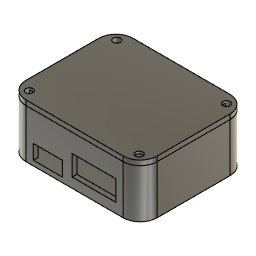
Box_motor (Autodesk Fusion 360 design; units mm, degrees)
Autodesk Fusion 360 part; units mm, degrees
sketch "Sketch1" plane through (0, 0, 0) normal (0, 0, 1) x (1, 0, 0)
  line L0 (-20, 20) -> (20, 20)
  line L1 (25, 15) -> (25, -15)
  line L2 (20, -20) -> (-20, -20)
  line L3 (-25, -15) -> (-25, 15)
  line L4 (-25, 20) -> (25, -20) construction
  line L5 (25, 20) -> (-25, -20) construction
  arc A0 (-25, -15) -> (-20, -20) centre (-20, -15) ccw
  arc A1 (-20, 20) -> (-25, 15) centre (-20, 15) ccw
  arc A2 (25, 15) -> (20, 20) centre (20, 15) ccw
  arc A3 (20, -20) -> (25, -15) centre (20, -15) ccw
  line L6 (20, -22) -> (-20, -22)
  arc A4 (-27, -15) -> (-20, -22) centre (-20, -15) ccw
  line L7 (-27, -15) -> (-27, 15)
  arc A5 (-20, 22) -> (-27, 15) centre (-20, 15) ccw
  line L8 (-20, 22) -> (20, 22)
  arc A6 (27, 15) -> (20, 22) centre (20, 15) ccw
  line L9 (27, 15) -> (27, -15)
  arc A7 (20, -22) -> (27, -15) centre (20, -15) ccw
  dimension "d1" = 50
  dimension "d2" = 40
  dimension "d3" = -2
  dimension "d4" = 5
  dimension "d5" = 5
  constraint horizontal L0
  constraint perpendicular L0 L1
  constraint parallel L0 L2
  constraint parallel L1 L3
  constraint coincident L4 origin
  constraint coincident L5 origin
  constraint coincident L5.end L3
  constraint coincident L5.end L2
  constraint tangent L3 A0
  constraint tangent L2 A0
  constraint coincident L4.start L3
  constraint coincident L4.start L0
  constraint tangent L3 A1
  constraint tangent L0 A1
  constraint equal A0 A1
  constraint coincident L5.start L1
  constraint coincident L5.start L0
  constraint tangent L1 A2
  constraint tangent L0 A2
  constraint coincident L4.end L1
  constraint coincident L4.end L2
  constraint tangent L1 A3
  constraint tangent L2 A3
  constraint equal A2 A3
  measures "d1" distance of L4.end L5.end
  measures "d2" distance of L5.start L4.end
  measures "d4" radius of A0
  measures "d5" radius of A2
extrude "Extrude1" add sketch "Sketch1" along normal blind 20 contours L0 L1 L2 L3 A0 A1 A2 A3 | L6 A4 L7 A5 L8 A6 L9 A7 makes body 1
shell "Shell1" thickness 2 removed faces 1 at (6.6667, -7.3333, 20) on bodies 1
sketch "Sketch2" plane through (0, -22, 0) normal (0, -1, 0) x (1, 0, 0)
  line L0 (-20, 0) -> (20, 0)
  line L1 (20, 0) -> (20, 20)
  line L2 (20, 20) -> (-20, 20)
  line L3 (-20, 20) -> (-20, 0)
  line L4 (-17, 8) -> (-5, 8)
  line L5 (-5, 8) -> (-5, 2)
  line L6 (-5, 2) -> (-17, 2)
  line L7 (-17, 2) -> (-17, 8)
  line L8 (-27, 0) -> (-27, 20)
  line L9 (-1, 2) -> (17, 2)
  line L10 (17, 2) -> (17, 12.4065)
  line L11 (17, 12.4065) -> (-1, 12.4065)
  line L12 (-1, 12.4065) -> (-1, 2)
  dimension "d9" = 10
  dimension "d10" = 12
  dimension "d11" = 2
  dimension "d12" = 6
  dimension "d13" = 2
  dimension "d14" = 4
  dimension "d15" = 18
  constraint horizontal L4
  constraint vertical L5
  constraint horizontal L6
  constraint vertical L7
  constraint horizontal L9
  constraint vertical L10
  constraint horizontal L11
  constraint vertical L12
  measures "d9" distance of L7 L8
  measures "d10" distance of L4.start L4.end
  measures "d11" distance of L0 L6
  measures "d12" distance of L4.end L5.end
  measures "d13" distance of L0 L9
  measures "d14" distance of L5 L12
  measures "d15" distance of L10.end L11.end
extrude "Extrude2" cut sketch "Sketch2" against normal blind 10 contours L4 L5 L6 L7 | L9 L10 L11 L12 bodies 1
sketch "Sketch3" plane through (0, 0, 20) normal (0, 0, 1) x (-1, 0, 0)
  line L0 (25, 15) -> (25, -15)
  arc A0 (20, -20) -> (25, -15) centre (20, -15) ccw
  line L1 (20, -20) -> (-20, -20)
  arc A1 (-25, -15) -> (-20, -20) centre (-20, -15) ccw
  line L2 (-25, -15) -> (-25, 15)
  arc A2 (-20, 20) -> (-25, 15) centre (-20, 15) ccw
  line L3 (-20, 20) -> (20, 20)
  arc A3 (25, 15) -> (20, 20) centre (20, 15) ccw
  arc A4 (27, 15) -> (20, 22) centre (20, 15) ccw
  line L4 (20, 22) -> (-20, 22)
  arc A5 (-20, 22) -> (-27, 15) centre (-20, 15) ccw
  line L5 (-27, 15) -> (-27, -15)
  arc A6 (-27, -15) -> (-20, -22) centre (-20, -15) ccw
  line L6 (-20, -22) -> (20, -22)
  arc A7 (20, -22) -> (27, -15) centre (20, -15) ccw
  line L7 (27, -15) -> (27, 15)
extrude "Extrude3" add sketch "Sketch3" along normal blind 2 separate body contours L0 A0 L1 A1 L2 A2 L3 A3 | A4 L4 A5 L5 A6 L6 A7 L7 makes body 2
extrude "Extrude4" add sketch "Sketch3" against normal blind 2 contours L0 A0 L1 A1 L2 A2 L3 A3 bodies 2
shell "Shell2" thickness 1 removed faces 1 at (6.6667, -6.6667, 18) on bodies 2
sketch "Sketch4" plane through (0, 0, 20) normal (0, 0, 1) x (-1, 0, 0)
  line L0 (25, 15) -> (25, -15)
  arc A0 (20, -20) -> (25, -15) centre (20, -15) ccw
  line L1 (20, -20) -> (-20, -20)
  arc A1 (-25, -15) -> (-20, -20) centre (-20, -15) ccw
  line L2 (-25, -15) -> (-25, 15)
  arc A2 (-20, 20) -> (-25, 15) centre (-20, 15) ccw
  line L3 (-20, 20) -> (20, 20)
  arc A3 (25, 15) -> (20, 20) centre (20, 15) ccw
  arc A4 (27, 15) -> (20, 22) centre (20, 15) ccw
  line L4 (20, 22) -> (-20, 22)
  arc A5 (-20, 22) -> (-27, 15) centre (-20, 15) ccw
  line L5 (-27, 15) -> (-27, -15)
  arc A6 (-27, -15) -> (-20, -22) centre (-20, -15) ccw
  line L6 (-20, -22) -> (20, -22)
  arc A7 (20, -22) -> (27, -15) centre (20, -15) ccw
  line L7 (27, -15) -> (27, 15)
  circle A8 centre (22.6, -18) radius 2.5
  circle A9 centre (22.6, -18) radius 0.75
  dimension "d23" = 5
  dimension "d24" = 1.5
  dimension "d35" = 18
  dimension "d36" = 22.6
  constraint concentric A8 A9
  measures "d23" diameter of A8
  measures "d24" diameter of A9
  measures "d35" vertical distance of origin A8.centre
  measures "d36" horizontal distance of origin A8.centre
extrude "Extrude5" add sketch "Sketch4" against normal blind 3.5 contours A0 A8 picked at (21.3866, -19.1562) bodies 1
mirror "Mirror1" about plane through (0, 0, 0) normal (1, 0, 0) of "Extrude5"
mirror "Mirror2" about plane through (0, 0, 0) normal (0, 1, 0) of "Extrude5", "Mirror1"
fillet "Fillet2" radius 1 8 edges at (-24.7143, 16.6659, 18.25) (-20.979, 19.9032, 18.25) (20.979, 19.9032, 18.25) (24.7143, 16.6659, 18.25) (-24.7143, -16.6659, 18.25) (-20.979, -19.9032, 18.25) (20.979, -19.9032, 18.25) (24.7143, -16.6659, 18.25) on bodies 1
sketch "Sketch5" plane through (0, 0, 22) normal (0, 0, 1) x (-1, 0, 0)
  line L0 (27, -15) -> (27, 15)
  arc A0 (27, 15) -> (20, 22) centre (20, 15) ccw
  line L1 (20, 22) -> (-20, 22)
  arc A1 (-20, 22) -> (-27, 15) centre (-20, 15) ccw
  line L2 (-27, 15) -> (-27, -15)
  arc A2 (-27, -15) -> (-20, -22) centre (-20, -15) ccw
  line L3 (-20, -22) -> (20, -22)
  arc A3 (20, -22) -> (27, -15) centre (20, -15) ccw
  circle A4 centre (22.6, -18) radius 1.5
  line L4 (0, 0) -> (0, -34.2644) construction
  dimension "d37" = 3
  dimension "d38" = 22.6
  dimension "d39" = 18
  constraint coincident L4.start origin
  constraint vertical L4
  measures "d37" diameter of A4
  measures "d38" horizontal distance of L4.start A4.centre
  measures "d39" vertical distance of L4.start A4.centre
extrude "Extrude6" cut sketch "Sketch5" against normal blind 4 contours A4 bodies 2
mirror "Mirror4" about plane through (0, 0, 0) normal (1, 0, 0) of "Extrude6"
mirror "Mirror5" about plane through (0, 0, 0) normal (0, 1, 0) of "Extrude6", "Mirror4"
fillet "Fillet3" radius 1.5 12 edges at (19.6229, -20, 16.5) (23.2747, -18.7784, 16.5) (25, -14.8961, 16.5) (-19.6229, 20, 16.5) (-23.2747, 18.7784, 16.5) (-25, 14.8961, 16.5) (-25, -14.8961, 16.5) (-23.2747, -18.7784, 16.5) (-19.6229, -20, 16.5) (25, 14.8961, 16.5) (23.2747, 18.7784, 16.5) (19.6229, 20, 16.5) on bodies 1
sketch "Sketch6" plane through (0, 0, 20) normal (0, 0, 1) x (-1, 0, 0)
  circle A0 centre (-22.6, 18) radius 0.75
  circle A1 centre (22.6, 18) radius 0.75
  circle A2 centre (-22.6, -18) radius 0.75
  circle A3 centre (22.6, -18) radius 0.75
  line L0 (25, 14.7922) -> (25, -14.7922)
  arc A4 (23.6, -15.7087) -> (25, -14.7922) centre (24, -14.7922) ccw
  arc A5 (23.6, -15.7087) -> (20.2042, -18.7143) centre (22.6, -18) ccw
  arc A6 (19.2459, -20) -> (20.2042, -18.7143) centre (19.2459, -19) ccw
  line L1 (19.2459, -20) -> (-19.2459, -20)
  arc A7 (-20.2042, -18.7143) -> (-19.2459, -20) centre (-19.2459, -19) ccw
  arc A8 (-20.2042, -18.7143) -> (-23.6, -15.7087) centre (-22.6, -18) ccw
  arc A9 (-25, -14.7922) -> (-23.6, -15.7087) centre (-24, -14.7922) ccw
  line L2 (-25, -14.7922) -> (-25, 14.7922)
  arc A10 (-23.6, 15.7087) -> (-25, 14.7922) centre (-24, 14.7922) ccw
  arc A11 (-23.6, 15.7087) -> (-20.2042, 18.7143) centre (-22.6, 18) ccw
  arc A12 (-19.2459, 20) -> (-20.2042, 18.7143) centre (-19.2459, 19) ccw
  line L3 (-19.2459, 20) -> (19.2459, 20)
  arc A13 (20.2042, 18.7143) -> (19.2459, 20) centre (19.2459, 19) ccw
  arc A14 (20.2042, 18.7143) -> (23.6, 15.7087) centre (22.6, 18) ccw
  arc A15 (25, 14.7922) -> (23.6, 15.7087) centre (24, 14.7922) ccw
  arc A16 (27, 15) -> (20, 22) centre (20, 15) ccw
  line L4 (20, 22) -> (-20, 22)
  arc A17 (-20, 22) -> (-27, 15) centre (-20, 15) ccw
  line L5 (-27, 15) -> (-27, -15)
  arc A18 (-27, -15) -> (-20, -22) centre (-20, -15) ccw
  line L6 (-20, -22) -> (20, -22)
  arc A19 (20, -22) -> (27, -15) centre (20, -15) ccw
  line L7 (27, -15) -> (27, 15)
  arc A20 (20, -22) -> (27, -15) centre (20, -15) ccw
  line L8 (-20, -22) -> (20, -22)
  line L9 (27, -15) -> (27, 15)
  arc A21 (27, 15) -> (20, 22) centre (20, 15) ccw
  line L10 (20, 22) -> (-20, 22)
  arc A22 (-20, 22) -> (-27, 15) centre (-20, 15) ccw
  line L11 (-27, 15) -> (-27, -15)
  arc A23 (-27, -15) -> (-20, -22) centre (-20, -15) ccw
  line L12 (25, -15) -> (25, 15)
  arc A24 (25, 15) -> (20, 20) centre (20, 15) ccw
  line L13 (20, 20) -> (-20, 20)
  arc A25 (-20, 20) -> (-25, 15) centre (-20, 15) ccw
  line L14 (-25, 15) -> (-25, -15)
  arc A26 (-25, -15) -> (-20, -20) centre (-20, -15) ccw
  line L15 (-20, -20) -> (20, -20)
  arc A27 (20, -20) -> (25, -15) centre (20, -15) ccw
  dimension "d50" = -2
extrude "Extrude7" cut sketch "Sketch6" against normal blind 1.5 contours A13 A14 A15 L12 A24 L13 | A4 A5 A6 L12 L15 A27 | A10 A11 A12 L13 A25 L14 | A7 A8 A9 L14 A26 L15 bodies 1
sketch "Sketch7" plane through (0, 0, 2) normal (0, 0, 1) x (-1, 0, 0)
  line L0 (-17, 20) -> (-20, 20)
  arc A0 (-20, 20) -> (-25, 15) centre (-20, 15) ccw
  line L1 (-25, 15) -> (-25, -15)
  arc A1 (-25, -15) -> (-20, -20) centre (-20, -15) ccw
  line L2 (-20, -20) -> (20, -20)
  arc A2 (20, -20) -> (25, -15) centre (20, -15) ccw
  line L3 (25, -15) -> (25, 15)
  arc A3 (25, 15) -> (20, 20) centre (20, 15) ccw
  line L4 (20, 20) -> (17, 20)
  line L5 (17, 20) -> (17, 22)
  line L6 (17, 22) -> (5, 22)
  line L7 (5, 22) -> (5, 20)
  line L8 (5, 20) -> (1, 20)
  line L9 (1, 20) -> (1, 22)
  line L10 (1, 22) -> (-17, 22)
  line L11 (-17, 22) -> (-17, 20)
  line L12 (1, 22) -> (-17, 22)
  line L13 (-17, 22) -> (-17, 20)
  line L14 (-17, 20) -> (1, 20)
  line L15 (1, 20) -> (1, 22)
  constraint horizontal L12
  constraint vertical L13
  constraint horizontal L14
  constraint vertical L15
  constraint coincident L0.start L11.end
  constraint coincident L9.end L10.start
extrude "Extrude8" add sketch "Sketch7" along normal blind 2 contours L9 L10 L11 L12 L13 L14 L15 bodies 1
named bodies: "Base", "Tapa"
